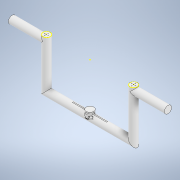
# Autodesk Inventor part: hands
Saved by Autodesk Inventor 2022 (Build 260153000, 153)
## iProperties
Created: 2023-06-18
Part Number: hands
Material: PVC-Piping
Document SubType Name: Modeling
Designer: jyoti
Density: 1.4 g/cm^3
Appearance: Smooth - White
Author: jyoti
Autodesk Inventor part; units mm, degrees
sketch "Sketch1" plane through (0, 0, 0) normal (0, 0, 1) x (1, 0, 0)
  line L0 (-126.3, 0) -> (126.3, 0)
  line L1 (126.3, 0) -> (126.3, 142.5)
  line L2 (126.3, 0) -> (268.8, 0) construction
  line L3 (-126.3, 0) -> (-126.3, 142.5)
  point P0 (0, 0)
  dimension "d0" = 252.6
  dimension "d1" = 142.5
  dimension "d2" = 90
  dimension "d3" = 142.5
  constraints: 8 end point, 2 coincident, 2 horizontal, 2 vertical, 1 perpendicular
  measures "d0" distance of L0.start L0.end
  measures "d1" distance of L0.end L1.end
  measures "d2" angle of L2 L1
  measures "d3" distance of L0.start L3.end
ref_plane "Work Plane1" through (-126.3, 142.5, 0) normal (0, 1, 0) x (-1, 0, 0)
sketch "Sketch2" plane through (-126.3, 142.5, 0) normal (0, 1, 0) x (-1, 0, 0)
  circle A0 centre (0, 0) radius 10.65
  point P0 (-126.3, 0)
  dimension "d4" = 21.3
  constraints: 1 centre point
  measures "d4" diameter of A0
sweep "Sweep1" add profiles "Sketch2" path "Sketch1"
ref_plane "Work Plane2" through (0, 0, 0) normal (0, 1, 0) x (-1, 0, 0)
sketch "Sketch3" plane through (0, 0, 0) normal (0, 1, 0) x (-1, 0, 0)
  circle A0 centre (0, 0) radius 11
  dimension "d8" = 22
  constraints: 1 centre point, 1 coincident
  measures "d8" diameter of A0
extrude "Extrusion1" add sketch "Sketch3" along normal blind 17.5
ref_plane "Work Plane3" through (0, 0, 0) normal (0, 0, 1) x (1, 0, 0)
sketch "Sketch4" plane through (0, 0, 0) normal (0, 0, 1) x (1, 0, 0)
  circle A0 centre (0, 12.5) radius 2.5
  point P0 (0, 0)
  dimension "d12" = 5
  constraints: 1 centre point
  measures "d12" diameter of A0
extrude "Extrusion2" cut sketch "Sketch4" along normal mid plane 100
ref_plane "Work Plane4" through (0, 0, 0) normal (1, 0, 0) x (0, 1, 0)
sketch "Sketch5" plane through (0, 0, 0) normal (1, 0, 0) x (0, 1, 0)
  circle A0 centre (12.5, 0) radius 2.5
  point P0 (0, 0)
  dimension "d16" = 5
  constraints: 1 centre point
  measures "d16" diameter of A0
extrude "Extrusion3" cut sketch "Sketch5" along normal mid plane 100
sketch "Sketch6" plane through (-126.3, 142.5, 0) normal (0, 1, 0) x (1, 0, 0)
  circle A0 centre (0, 0) radius 10.65 projected
  point P0 (126.3, 0)
  constraints: 1 coincident
sketch "Sketch7" plane through (126.3, 142.5, 0) normal (0, 1, 0) x (1, 0, 0)
  circle A0 centre (0, 0) radius 10.65 projected
  point P0 (-126.3, 0)
  constraints: 1 coincident
ref_plane "Work Plane6" through (126.3, 0, 0) normal (1, 0, 0) x (0, 1, 0)
ref_plane "Work Plane7" through (-126.3, 0, 0) normal (1, 0, 0) x (0, 1, 0)
sketch "Sketch8" plane through (-126.3, 0, 0) normal (1, 0, 0) x (0, 1, 0)
  line L0 (142.5, -10.65) -> (142.5, 10.65) projected
  circle A0 centre (130, 0) radius 10.65
  point P0 (0, 0)
  point P1 (142.5, 0)
  dimension "d21" = 21.3
  constraints: 1 centre point, 1 midpoint
  measures "d21" diameter of A0
extrude "Extrusion4" add sketch "Sketch8" against normal blind 100
sketch "Sketch9" plane through (126.3, 0, 0) normal (1, 0, 0) x (0, 1, 0)
  circle A0 centre (130, 0) radius 10.65 projected
  circle A1 centre (130, 0) radius 10.65
  point P0 (0, 0)
  constraints: 1 centre point, 1 coincident
extrude "Extrusion5" add sketch "Sketch9" along normal blind 100
body "Solid1"
